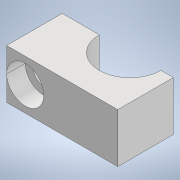
# Autodesk Inventor part: Extruder Cable Clamp
Saved by Autodesk Inventor 2020 (Build 240168000, 168)
## iProperties
Created: 2019-11-15
Part Number: Extruder Cable Clamp
Material: Generic
Document SubType Name: Modeling
Designer: pepd9
Density: 1 g/cm^3
Appearance: Default
Author: pepd9
Autodesk Inventor part; units mm, degrees
ref_plane "YZ Plane" through (0, 0, 0) normal (1, 0, 0) x (0, 1, 0)
ref_plane "XZ Plane" through (0, 0, 0) normal (0, 1, 0) x (-1, 0, 0)
ref_plane "XY Plane" through (0, 0, 0) normal (0, 0, 1) x (1, 0, 0)
sketch "Sketch1" plane through (0, 0, 0) normal (0, 1, 0) x (-1, 0, 0)
  arc A0 (-10, 0) -> (0, 0) centre (-5, 0) ccw projected
  line L0 (6, 0) -> (0, 0) projected
  line L1 (-10, 0) -> (-12, 0) projected
  circle A1 centre (-5, 0) radius 5
  line L2 (-12, 0) -> (6, 0)
  line L3 (6, 0) -> (6, 9)
  line L4 (6, 9) -> (-12, 9)
  line L5 (-12, 9) -> (-12, 0)
  point P0 (0, 0)
  dimension "d0" = 9
  constraints: 8 end point, 2 parallel, 1 coincident, 1 horizontal, 1 perpendicular, 1 point on line, 3 other
  measures "d0" distance of L2.end L3.end
ref_plane "Work Plane1" through (-6, -8, -5) normal (0, -1, 0) x (1, 0, 0)
extrude "Extrusion1" add sketch "Sketch1" against normal up to surface (8 mm away) contours L1 L5 L4 L3 L0 A1
sketch "Sketch2" plane through (-6, 0, 9) normal (0, 0, 1) x (1, 0, 0)
  circle A0 centre (3.5, -4) radius 1.7 projected
  point P0 (3, -4)
hole "Hole1" at (-2.5, -4, 9) direction (0, 0, -1) diameter 3.4 end through all counterbore diameter 6 counterbore depth 3
fillet "Fillet1" radius 8 1 edges at (12, -4, 9)
fillet "Fillet2" radius 5.5 1 edges at (-6, -4, 9)
ref_plane "Work Plane2" through (5, -7.5, 0) normal (0, -1, 0) x (1, 0, 0)
sketch "Sketch3" plane through (5, -7.5, 0) normal (0, -1, 0) x (1, 0, 0)
  arc A0 (5, 0) -> (-5, 0) centre (0, 0) ccw projected
  circle A1 centre (0, 0) radius 4.5
  line L0 (-5, 0) -> (-4.5, 0)
  line L1 (-4.8547, 1.1966) -> (-4.3692, 1.0769)
  line L2 (-4.4273, 2.3236) -> (-3.9846, 2.0913)
  line L3 (-3.7426, 3.3156) -> (-3.3683, 2.9841)
  line L4 (-2.8403, 4.1149) -> (-2.5563, 3.7034)
  line L5 (-1.773, 4.6751) -> (-1.5957, 4.2076)
  line L6 (-0.6027, 4.9635) -> (-0.5424, 4.4672)
  line L7 (0.6027, 4.9635) -> (0.5424, 4.4672)
  line L8 (1.773, 4.6751) -> (1.5957, 4.2076)
  line L9 (2.8403, 4.1149) -> (2.5563, 3.7034)
  line L10 (3.7426, 3.3156) -> (3.3683, 2.9841)
  line L11 (4.4273, 2.3236) -> (3.9846, 2.0913)
  line L12 (4.8547, 1.1966) -> (4.3692, 1.0769)
  line L13 (5, 0) -> (4.5, 0)
  point P0 (-3.9846, 2.0913)
  point P1 (-4.4273, 2.3236)
  point P2 (-2.5563, 3.7034)
  point P3 (-2.8403, 4.1149)
  point P4 (-3.7426, 3.3156)
  point P5 (-3.3683, 2.9841)
  point P6 (-0.5424, 4.4672)
  point P7 (-1.5957, 4.2076)
  point P8 (1.5957, 4.2076)
  point P9 (1.773, 4.6751)
  point P10 (0.6027, 4.9635)
  point P11 (0.5424, 4.4672)
  point P12 (3.3683, 2.9841)
  point P13 (3.7426, 3.3156)
  point P14 (2.8403, 4.1149)
  point P15 (2.5563, 3.7034)
  point P16 (3.9846, 2.0913)
  dimension "d13" = 9
  dimension "d16" = 180
  constraints: 28 end point, 1 coincident, 1 horizontal, 43 other
extrude "Extrusion2" add sketch "Sketch3" against normal blind 0.75 contours L12 A1 L11 A0 | L10 A1 L9 A0 | L1 A0 L2 A1 | L8 A1 L7 A0 | L3 A0 L4 A1 | L6 A1 L5 A0
pattern_linear "Rectangular Pattern1" count 4 spacing 2 along (0, 1, 0) of "Extrusion2"
body "Solid1"
